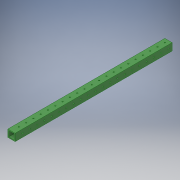
# Autodesk Inventor part: Kermit Frame 11
Saved by Autodesk Inventor 2018.2 (Build 222227000, 227)
## iProperties
Created: 2018-02-06
Part Number: Kermit Frame 11
Material: Generic
Document SubType Name: Modeling
Designer: lopez.xavier
Density: 1 g/cm^3
Appearance: Smooth - Dark Forest Green
Author: lopez.xavier
Autodesk Inventor part; units mm, degrees
ref_plane "YZ Plane" through (0, 0, 0) normal (1, 0, 0) x (0, 1, 0)
ref_plane "XZ Plane" through (0, 0, 0) normal (0, 1, 0) x (-1, 0, 0)
ref_plane "XY Plane" through (0, 0, 0) normal (0, 0, 1) x (1, 0, 0)
sketch "Sketch1" plane through (0, 0, 0) normal (0, 0, 1) x (1, 0, 0)
  line L0 (0, 0) -> (25.4, 0)
  line L1 (25.4, 0) -> (25.4, 25.4)
  line L2 (25.4, 25.4) -> (0, 25.4)
  line L3 (0, 25.4) -> (0, 0)
  dimension "d0" = 25.4
  dimension "d1" = 25.4
  constraints: 8 end point, 2 parallel, 1 horizontal, 1 perpendicular
  measures "d0" distance of L2.end L1.end
  measures "d1" distance of L1.end L0.end
extrude "Extrusion1" add sketch "Sketch1" along normal blind 546.1
shell "Shell1" thickness 3.175 removed faces 2 at (8.4667, 16.9333, 0) at (8.4667, 16.9333, 546.1)
sketch "Sketch2" plane through (25.4, 0, 0) normal (1, 0, 0) x (0, 0, -1)
  circle A0 centre (-12.7, 12.7) radius 1.9685
  line L0 (0, 25.4) -> (-546.1, 25.4) projected
  line L1 (0, 0) -> (0, 25.4) projected
  circle A1 centre (-38.1, 12.7) radius 1.9685
  circle A2 centre (-63.5, 12.7) radius 1.9685
  circle A3 centre (-88.9, 12.7) radius 1.9685
  circle A4 centre (-114.3, 12.7) radius 1.9685
  circle A5 centre (-139.7, 12.7) radius 1.9685
  circle A6 centre (-165.1, 12.7) radius 1.9685
  circle A7 centre (-190.5, 12.7) radius 1.9685
  circle A8 centre (-215.9, 12.7) radius 1.9685
  circle A9 centre (-241.3, 12.7) radius 1.9685
  circle A10 centre (-266.7, 12.7) radius 1.9685
  circle A11 centre (-292.1, 12.7) radius 1.9685
  circle A12 centre (-317.5, 12.7) radius 1.9685
  circle A13 centre (-342.9, 12.7) radius 1.9685
  circle A14 centre (-368.3, 12.7) radius 1.9685
  circle A15 centre (-393.7, 12.7) radius 1.9685
  circle A16 centre (-419.1, 12.7) radius 1.9685
  circle A17 centre (-444.5, 12.7) radius 1.9685
  circle A18 centre (-469.9, 12.7) radius 1.9685
  circle A19 centre (-495.3, 12.7) radius 1.9685
  circle A20 centre (-520.7, 12.7) radius 1.9685
  dimension "d5" = 3.937
  dimension "d6" = 12.7
  dimension "d7" = 12.7
  dimension "d10" = 25.4
  constraints: 21 centre point, 1 horizontal, 40 other
  measures "d5" diameter of A0
  measures "d6" distance from line of L0 A0.centre
  measures "d7" distance from line of L1 A0.centre
  measures "d10" distance of A0.centre A1.centre
extrude "Extrusion2" cut sketch "Sketch2" against normal blind 542.925
sketch "Sketch3" plane through (0, 25.4, 0) normal (0, 1, 0) x (1, 0, 0)
  circle A0 centre (12.7, -12.7) radius 1.9685
  line L0 (0, 0) -> (0, -546.1) projected
  line L1 (25.4, 0) -> (0, 0) projected
  circle A1 centre (12.7, -38.1) radius 1.9685
  circle A2 centre (12.7, -63.5) radius 1.9685
  circle A3 centre (12.7, -88.9) radius 1.9685
  circle A4 centre (12.7, -114.3) radius 1.9685
  circle A5 centre (12.7, -139.7) radius 1.9685
  circle A6 centre (12.7, -165.1) radius 1.9685
  circle A7 centre (12.7, -190.5) radius 1.9685
  circle A8 centre (12.7, -215.9) radius 1.9685
  circle A9 centre (12.7, -241.3) radius 1.9685
  circle A10 centre (12.7, -266.7) radius 1.9685
  circle A11 centre (12.7, -292.1) radius 1.9685
  circle A12 centre (12.7, -317.5) radius 1.9685
  circle A13 centre (12.7, -342.9) radius 1.9685
  circle A14 centre (12.7, -368.3) radius 1.9685
  circle A15 centre (12.7, -393.7) radius 1.9685
  circle A16 centre (12.7, -419.1) radius 1.9685
  circle A17 centre (12.7, -444.5) radius 1.9685
  circle A18 centre (12.7, -469.9) radius 1.9685
  circle A19 centre (12.7, -495.3) radius 1.9685
  circle A20 centre (12.7, -520.7) radius 1.9685
  dimension "d17" = 3.937
  dimension "d18" = 12.7
  dimension "d19" = 12.7
  dimension "d22" = 25.4
  constraints: 21 centre point, 1 vertical, 40 other
  measures "d17" diameter of A0
  measures "d18" distance from line of L0 A0.centre
  measures "d19" distance from line of L1 A0.centre
  measures "d22" distance of A0.centre A1.centre
extrude "Extrusion3" cut sketch "Sketch3" against normal blind 542.925
body "Solid1"
